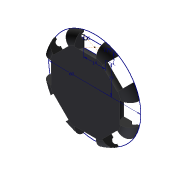
# Autodesk Inventor part: omni_wheel_cover_out_v3
Saved by Autodesk Inventor 2017 (Build 210142000, 142)
## iProperties
Created: 2018-10-27
Part Number: omni_wheel_cover_out_v3
Material: Generic
Document SubType Name: Modeling
Designer: mfans
Density: 1 g/cm^3
Appearance: Default
Author: mfans
Autodesk Inventor part; units mm, degrees
ref_plane "YZ Plane" through (0, 0, 0) normal (1, 0, 0) x (0, 1, 0)
ref_plane "XZ Plane" through (0, 0, 0) normal (0, 1, 0) x (-1, 0, 0)
ref_plane "XY Plane" through (0, 0, 0) normal (0, 0, 1) x (1, 0, 0)
sketch "Sketch1" plane through (0, 0, 0) normal (0, 1, 0) x (-1, 0, 0)
  circle A0 centre (0, 0) radius 30
  line L0 (7, 26) -> (-7, 26)
  line L1 (-7, 26) -> (-7, 19)
  line L2 (-7, 19) -> (7, 19)
  line L3 (7, 19) -> (7, 26)
  line L4 (7, 26) -> (-7, 19) construction
  line L5 (-7, 26) -> (7, 19) construction
  line L6 (7, 24.25) -> (8.7854, 24.25)
  line L7 (-7, 24.25) -> (-8.7854, 24.25)
  line L8 (9.5, 26) -> (-9.5, 26)
  arc A1 (4.5, 26) -> (7, 23.5) centre (7, 26) ccw
  arc A2 (8.7854, 24.25) -> (9.5, 26) centre (7, 26) ccw
  arc A3 (-9.5, 26) -> (-8.7854, 24.25) centre (-7, 26) ccw
  arc A4 (-7, 23.5) -> (-4.5, 26) centre (-7, 26) ccw
  point P0 (0, 22.5)
  dimension "d0" = 60
  dimension "d1" = 14
  dimension "d2" = 7
  dimension "d3" = 19
  dimension "d6" = 1.75
  dimension "d7" = 1.75
  constraints: 18 end point, 8 point on circle, 6 point on line, 5 centre point, 3 coincident, 3 horizontal, 2 midpoint, 2 parallel, 2 perpendicular
  measures "d0" diameter of A0
  measures "d1" distance of L2.end L1.end
  measures "d2" distance of L0.end L1.end
  measures "d3" distance from line of point (0, 0) L2
  measures "d6" distance between parallel lines of L0 L6
  measures "d7" distance between parallel lines of L0 L7
extrude "Extrusion1" add sketch "Sketch1" against normal blind 6 contours A0 | L3 A1 L0 | L8 A2 L6 L3 | A1 L3 L2 L1 A4 L0 | A4 L1 L0 | L1 L7 A3 L8
revolve "Revolution1" cut sketch "Sketch1" angle 360 about axis through (-7, 0, 26) along (1, 0, 0) contours L3 A1 L0 | L8 A2 L6 L3 | A1 L3 L2 L1 A4 L0 | A4 L1 L0 | L1 L7 A3 L8
sketch "Sketch2" plane through (0, -6, 0) normal (0, -1, 0) x (1, 0, 0)
  line L0 (-4.8488, 29.6056) -> (4.8488, 29.6056) projected
  arc A0 (4.8488, 29.6056) -> (-4.8488, 29.6056) centre (0, 0) ccw projected
extrude "Extrusion2" cut sketch "Sketch2" against normal blind 12
fillet "Fillet1" radius 6 1 edges at (0, -6, -30)
pattern_circular "Circular Pattern1" count 8 over 360 about axis through (0, -10, 0) along (0, 1, 0) of "Revolution1", "Extrusion2"
body "Solid1"
